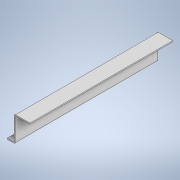
# Autodesk Inventor part: crossPlate
Saved by Autodesk Inventor 2020.2 (Build 242310000, 310)
## iProperties
Created: 2020-01-12
Part Number: crossPlate
Material: Generic
Document SubType Name: Modeling
Designer: robst
Density: 1 g/cm^3
Appearance: Default
Author: robst
Autodesk Inventor part; units mm, degrees
ref_plane "YZ Plane" through (0, 0, 0) normal (1, 0, 0) x (0, 1, 0)
ref_plane "XZ Plane" through (0, 0, 0) normal (0, 1, 0) x (-1, 0, 0)
ref_plane "XY Plane" through (0, 0, 0) normal (0, 0, 1) x (1, 0, 0)
sketch "Sketch1" plane through (0, 0, 0) normal (0, 0, 1) x (1, 0, 0)
  line L0 (0, 0) -> (19.05, 0)
  line L1 (22.225, 3.175) -> (22.225, 68.199)
  line L2 (22.225, 68.199) -> (63.5, 68.199)
  line L3 (63.5, 68.199) -> (63.5, 71.374)
  line L4 (63.5, 71.374) -> (22.9616, 71.374)
  line L5 (19.05, 67.4624) -> (19.05, 3.175)
  line L6 (19.05, 3.175) -> (0, 3.175)
  line L7 (0, 3.175) -> (0, 0)
  arc A0 (19.05, 0) -> (22.225, 3.175) centre (19.05, 3.175) ccw
  arc A1 (22.9616, 71.374) -> (19.05, 67.4624) centre (22.9616, 67.4624) ccw
  point P0 (22.225, 0)
  point P1 (19.05, 71.374)
  dimension "d0" = 22.225
  dimension "d1" = 68.199
  dimension "d2" = 41.275
  dimension "d3" = 3.175
  dimension "d4" = 44.45
  dimension "d5" = 68.199
  dimension "d6" = 3.175
  dimension "d7" = 3.9116
  constraints: 16 end point, 6 perpendicular, 4 point on circle, 4 point on line, 4 tangent, 2 centre point, 1 horizontal, 1 parallel
  measures "d0" distance of L0.start point (22.225, 0)
  measures "d1" distance of point (22.225, 0) L1.end
  measures "d2" distance of L1.end L2.end
  measures "d3" distance of L2.end L3.end
  measures "d4" distance of L3.end point (19.05, 71.374)
  measures "d5" distance of point (19.05, 71.374) L5.end
  measures "d6" radius of A0
  measures "d7" radius of A1
extrude "Extrusion1" add sketch "Sketch1" along normal mid plane 400.05
body "Solid1"
